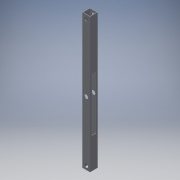
# Autodesk Inventor part: AP 5
Saved by Autodesk Inventor 2016 (Build 200138000, 138)
## iProperties
Created: 2016-02-17
Part Number: AP 5
Material: Generic
Document SubType Name: Modeling
Designer: Admin
Density: 1 g/cm^3
Appearance: Default
Author: Admin
Autodesk Inventor part; units mm, degrees
ref_plane "YZ Plane" through (0, 0, 0) normal (1, 0, 0) x (0, 1, 0)
ref_plane "XZ Plane" through (0, 0, 0) normal (0, 1, 0) x (-1, 0, 0)
ref_plane "XY Plane" through (0, 0, 0) normal (0, 0, 1) x (1, 0, 0)
sketch "Sketch1" plane through (0, 0, 0) normal (0, 1, 0) x (-1, 0, 0)
  line L0 (0, 0) -> (25.4, 0)
  line L1 (25.4, 0) -> (25.4, -25.4)
  line L2 (25.4, -25.4) -> (0, -25.4)
  line L3 (0, -25.4) -> (0, 0)
  line L4 (23.8125, -23.8125) -> (23.8125, -1.5875)
  line L5 (23.8125, -1.5875) -> (1.5875, -1.5875)
  line L6 (1.5875, -1.5875) -> (1.5875, -23.8125)
  line L7 (1.5875, -23.8125) -> (23.8125, -23.8125)
  dimension "d0" = 25.4
  dimension "d1" = 25.4
  dimension "d2" = 1.5875
  constraints: 16 end point, 4 parallel, 2 perpendicular, 1 horizontal, 3 other
  measures "d0" distance of L1.end L2.end
  measures "d1" distance of L0.end L1.end
  measures "d2" distance between parallel lines of L1 L4
extrude "Extrusion1" add sketch "Sketch1" along normal blind 444.5
sketch "Sketch2" plane through (-25.4, 0, 0) normal (0, 0, 1) x (1, 0, 0)
  circle A0 centre (12.7, 431.8) radius 6.35
  line L0 (0, 444.5) -> (25.4, 444.5) projected
  point P0 (25.4, 0)
  dimension "d5" = 12.7
  dimension "d6" = 12.7
  constraints: 1 centre point
  measures "d5" diameter of A0
  measures "d6" distance from line of L0 A0.centre
extrude "Extrusion2" cut sketch "Sketch2" against normal blind 25.4
sketch "Sketch4" plane through (0, 0, -25.4) normal (0, 0, -1) x (-1, 0, 0)
  circle A0 centre (12.7, 12.7) radius 6.35
  line L0 (25.4, 0) -> (0, 0) projected
  line L1 (0, 0) -> (0, 444.5) projected
  dimension "d17" = 12.7
  dimension "d18" = 12.7
  dimension "d19" = 12.7
  constraints: 1 centre point
  measures "d17" diameter of A0
  measures "d18" distance from line of L0 A0.centre
  measures "d19" distance from line of L1 A0.centre
extrude "Extrusion4" cut sketch "Sketch4" against normal blind 25.4
sketch "Sketch5" plane through (0, 0, -25.4) normal (0, 0, -1) x (-1, 0, 0)
  circle A0 centre (12.7, 209.55) radius 6.35
  line L0 (0, 0) -> (0, 444.5) projected
  line L1 (0, 444.5) -> (25.4, 444.5) projected
  dimension "d22" = 12.7
  dimension "d23" = 12.7
  dimension "d24" = 234.95
  constraints: 1 centre point
  measures "d22" diameter of A0
  measures "d23" distance from line of L0 A0.centre
  measures "d24" distance from line of L1 A0.centre
extrude "Extrusion5" cut sketch "Sketch5" against normal blind 25.4
sketch "Sketch6" plane through (0, 0, 0) normal (1, 0, 0) x (0, 0, -1)
  line L0 (5.08, 265.303) -> (20.32, 265.303)
  line L1 (20.32, 265.303) -> (20.32, 88.9)
  line L2 (20.32, 88.9) -> (5.08, 88.9)
  line L3 (5.08, 88.9) -> (5.08, 265.303)
  line L4 (23.8125, 444.5) -> (1.5875, 444.5) projected
  line L5 (25.4, 0) -> (25.4, 444.5) projected
  line L6 (0, 0) -> (0, 444.5) projected
  line L7 (25.4, 0) -> (0, 0) projected
  dimension "d28" = 5.08
  dimension "d29" = 5.08
  dimension "d30" = 176.403
  dimension "d33" = 88.9
  constraints: 8 end point, 2 parallel, 1 horizontal, 1 perpendicular
  measures "d28" distance between parallel lines of L5 L1
  measures "d29" distance between parallel lines of L6 L3
  measures "d30" distance of L0.end L1.end
  measures "d33" distance between parallel lines of L2 L7
extrude "Extrusion6" cut sketch "Sketch6" against normal blind 25.4
body "Solid1"
